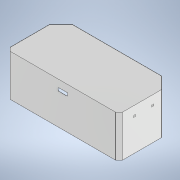
# Autodesk Inventor part: Carcasa
Saved by Autodesk Inventor 2022.1 (Build 261234000, 234)
## iProperties
Created: 2021-10-13
Part Number: Carcasa
Material: PVC, no plastificado
Document SubType Name: Modeling
Designer: seb_0
Density: 1.29 g/cm^3
Appearance: Suave - Blanco
Author: seb_0
Autodesk Inventor part; units mm, degrees
ref_plane "YZ Plane" through (0, 0, 0) normal (1, 0, 0) x (0, 1, 0)
ref_plane "XZ Plane" through (0, 0, 0) normal (0, 1, 0) x (-1, 0, 0)
ref_plane "Plano de trabajo1" through (0, 15.93, 0) normal (0, 0, 1) x (1, 0, 0)
sketch "Boceto1" plane through (0, 15.93, 0) normal (0, 0, 1) x (1, 0, 0)
  line L0 (225, 372.2908) -> (225, -4.1508) projected
  line L1 (224.6622, -4.9663) -> (193.0363, -36.5922) projected
  line L2 (113.0363, 484.7322) -> (224.6622, 373.1063) projected
  line L3 (-744.2208, 485.07) -> (112.2208, 485.07) projected
  line L4 (-857, -4.1508) -> (-857, 372.2908) projected
  line L5 (-825.0363, -36.5922) -> (-856.6622, -4.9663) projected
  line L6 (-856.6622, 373.1063) -> (-745.0363, 484.7322) projected
  line L7 (224.6622, 373.1063) -> (225, 372.2908)
  line L8 (112.2208, 485.07) -> (113.0363, 484.7322)
  line L9 (225, -4.1508) -> (224.6622, -4.9663)
  line L10 (192.2208, -36.93) -> (-824.2208, -36.93) projected
  line L11 (192.2208, -36.93) -> (193.0363, -36.5922)
  line L12 (-825.0363, -36.5922) -> (-824.2208, -36.93)
  line L13 (-857, -4.1508) -> (-856.6622, -4.9663)
  line L14 (-857, 372.2908) -> (-856.6622, 373.1063)
  line L15 (-745.0363, 484.7322) -> (-744.2208, 485.07)
  line L16 (-858.5, -4.4491) -> (-860.9339, 1.4267)
  line L17 (-824.5191, -38.43) -> (192.5191, -38.43)
  line L18 (192.5191, -38.43) -> (193.886, -37.8639)
  line L19 (193.886, -37.8639) -> (225.9339, -5.816)
  line L20 (225.9339, -5.816) -> (226.5, -4.4491)
  line L21 (226.5, -4.4491) -> (226.5, 372.5891)
  line L22 (226.5, 372.5891) -> (225.9339, 373.956)
  line L23 (225.9339, 373.956) -> (113.886, 486.0039)
  line L24 (113.886, 486.0039) -> (112.5191, 486.57)
  line L25 (112.5191, 486.57) -> (-744.5191, 486.57)
  line L26 (-744.5191, 486.57) -> (-745.886, 486.0039)
  line L27 (-745.886, 486.0039) -> (-857.9339, 373.956)
  line L28 (-857.9339, 373.956) -> (-858.5, 372.5891)
  line L29 (-858.5, 372.5891) -> (-858.5, -4.4491)
  line L30 (-858.5, -4.4491) -> (-857.9339, -5.816)
  line L31 (-857.9339, -5.816) -> (-825.886, -37.8639)
  line L32 (-825.886, -37.8639) -> (-824.5191, -38.43)
  point P0 (0, -15.93)
  dimension "d63" = 1.5
  constraints: 50 end point, 8 perpendicular, 15 other
  measures "d63" distance between parallel lines of L10 L17
extrude "Extrusión1" add sketch "Boceto1" against normal blind 400
sketch "Boceto2" plane through (0, 15.93, 0) normal (0, 0, 1) x (1, 0, 0)
  line L0 (-857, -4.1508) -> (-857, 372.2908)
  line L1 (-857, 372.2908) -> (-856.6622, 373.1063)
  line L2 (-856.6622, 373.1063) -> (-745.0363, 484.7322)
  line L3 (-745.0363, 484.7322) -> (-744.2208, 485.07)
  line L4 (-744.2208, 485.07) -> (112.2208, 485.07)
  line L5 (112.2208, 485.07) -> (113.0363, 484.7322)
  line L6 (113.0363, 484.7322) -> (224.6622, 373.1063)
  line L7 (224.6622, 373.1063) -> (225, 372.2908)
  line L8 (225, 372.2908) -> (225, -4.1508)
  line L9 (225, -4.1508) -> (224.6622, -4.9663)
  line L10 (224.6622, -4.9663) -> (193.0363, -36.5922)
  line L11 (-825.0363, -36.5922) -> (-856.6622, -4.9663)
  line L12 (-825.0363, -36.5922) -> (-856.6622, -4.9663)
  line L13 (224.6622, -4.9663) -> (193.0363, -36.5922)
  line L14 (192.2208, -36.93) -> (-824.2208, -36.93)
  line L15 (-857, -4.1508) -> (-857, 372.2908)
  line L16 (193.0363, -36.5922) -> (192.2208, -36.93)
  line L17 (192.2208, -36.93) -> (-824.2208, -36.93)
  line L18 (-824.2208, -36.93) -> (-825.0363, -36.5922)
  line L19 (-825.0363, -36.5922) -> (-856.6622, -4.9663)
  line L20 (-856.6622, -4.9663) -> (-857, -4.1508)
  line L21 (112.5191, 486.57) -> (-744.5191, 486.57)
  line L22 (-825.886, -37.8639) -> (-824.5191, -38.43)
  line L23 (-824.5191, -38.43) -> (192.5191, -38.43)
  line L24 (192.5191, -38.43) -> (193.886, -37.8639)
  line L25 (193.886, -37.8639) -> (225.9339, -5.816)
  line L26 (225.9339, -5.816) -> (226.5, -4.4491)
  line L27 (226.5, -4.4491) -> (226.5, 372.5891)
  line L28 (226.5, 372.5891) -> (225.9339, 373.956)
  line L29 (225.9339, 373.956) -> (113.886, 486.0039)
  line L30 (113.886, 486.0039) -> (112.5191, 486.57)
  line L31 (112.5191, 486.57) -> (-744.5191, 486.57)
  line L32 (-744.5191, 486.57) -> (-745.886, 486.0039)
  line L33 (-745.886, 486.0039) -> (-857.9339, 373.956)
  line L34 (-857.9339, 373.956) -> (-858.5, 372.5891)
  line L35 (-858.5, 372.5891) -> (-858.5, -4.4491)
  line L36 (-858.5, -4.4491) -> (-857.9339, -5.816)
  line L37 (-857.9339, -5.816) -> (-825.886, -37.8639)
  line L38 (-857, -4.1508) -> (-857, 372.2908)
  line L39 (-857, 372.2908) -> (-856.6622, 373.1063)
  line L40 (-856.6622, 373.1063) -> (-745.0363, 484.7322)
  line L41 (-745.0363, 484.7322) -> (-744.2208, 485.07)
  line L42 (-744.2208, 485.07) -> (112.2208, 485.07)
  line L43 (112.2208, 485.07) -> (113.0363, 484.7322)
  line L44 (113.0363, 484.7322) -> (224.6622, 373.1063)
  line L45 (224.6622, 373.1063) -> (225, 372.2908)
  line L46 (225, 372.2908) -> (225, -4.1508)
  line L47 (225, -4.1508) -> (224.6622, -4.9663)
  line L48 (224.6622, -4.9663) -> (193.0363, -36.5922)
  line L49 (193.0363, -36.5922) -> (192.2208, -36.93)
  line L50 (192.2208, -36.93) -> (-824.2208, -36.93)
  line L51 (-824.2208, -36.93) -> (-825.0363, -36.5922)
  line L52 (-825.0363, -36.5922) -> (-856.6622, -4.9663)
  line L53 (-856.6622, -4.9663) -> (-857, -4.1508)
  point P0 (-824.2208, -36.93)
extrude "Extrusión2" add sketch "Boceto2" along normal blind 1.5 contours L0 L1 L2 L3 L4 L5 L6 L7 L8 L9 L10 L16 L14 L18 L11 L20 | L30 L29 L28 L27 L26 L25 L24 L23 L22 L37 L36 L35 L34 L33 L32 L21
sketch "Boceto4" plane through (-744.5191, 502.5, -400) normal (0, 1, 0) x (1, 0, 0)
  line L0 (855.1466, -300) -> (1.8917, -300) projected
  circle A0 centre (655.1466, -310) radius 2.5
  circle A1 centre (201.8917, -310) radius 2.5
  point P0 (744.5191, -400)
  dimension "d5" = 10
  dimension "d6" = 10
  dimension "d7" = 5
  dimension "d8" = 200
  dimension "d9" = 200
  constraints: 2 centre point, 1 equal radius
  measures "d5" distance from line of L0 A0.centre
  measures "d6" distance from line of L0 A1.centre
  measures "d7" diameter of A0
  measures "d8" horizontal distance of L0.start A0.centre
  measures "d9" horizontal distance of A1.centre L0.end
hole "Agujero1" at (-89.3726, 502.5, -90) at (-542.6274, 502.5, -90) direction (0, -1, 0) diameter 3.4 depth 6 tip angle 118 clearance for "Tornillo para maquinaria de cabeza plana" size "M3" standard "Perfil M métrico ANSI"
sketch "Boceto6" plane through (-744.2208, 501, -400) normal (0, -1, 0) x (1, 0, 0)
  circle A0 centre (654.8482, 310) radius 1.7 projected
  circle A1 centre (201.5934, 310) radius 1.7 projected
  circle A2 centre (654.8482, 310) radius 9.2
  circle A3 centre (201.5934, 310) radius 9.2
  line L0 (664.0482, 300.8) -> (645.6482, 300.8)
  line L1 (645.6482, 300.8) -> (645.6482, 319.2)
  line L2 (645.6482, 319.2) -> (664.0482, 319.2)
  line L3 (664.0482, 319.2) -> (664.0482, 300.8)
  line L4 (210.7934, 300.8) -> (192.3934, 300.8)
  line L5 (192.3934, 300.8) -> (192.3934, 319.2)
  line L6 (192.3934, 319.2) -> (210.7934, 319.2)
  line L7 (210.7934, 319.2) -> (210.7934, 300.8)
  point P0 (744.2208, 400)
  dimension "d17" = 7.5
  constraints: 16 end point, 8 tangent, 4 parallel, 2 centre point, 2 horizontal, 2 perpendicular, 1 equal radius
  measures "d17" radial gap between concentric circles of A0 A2
extrude "Extrusión3" add sketch "Boceto6" along normal blind 15
sketch "Boceto7" plane through (-858.5, 27.4109, -400) normal (-1, 0, 0) x (0, 0, 1)
  line L0 (264, 376.8034) -> (264, 0.2349) projected
  circle A0 centre (310, 276.8034) radius 2.5
  circle A1 centre (310, 100.2349) radius 2.5
  line L1 (300, 359.2166) -> (300, -14.0383) projected
  point P0 (400, -27.4109)
  dimension "d21" = 5
  dimension "d23" = 100
  dimension "d24" = 100
  dimension "d60" = 10
  dimension "d62" = 10
  constraints: 2 centre point, 1 equal radius
  measures "d21" diameter of A0
  measures "d23" vertical distance of L0.start A0.centre
  measures "d24" vertical distance of L0.end A1.centre
  measures "d60" distance from line of L1 A0.centre
  measures "d62" distance from line of L1 A1.centre
hole "Agujero2" at (-858.5, 304.2143, -90) at (-858.5, 127.6457, -90) direction (1, 0, 0) diameter 3.4 end through all clearance for "Tornillo para maquinaria de cabeza plana" size "M3" standard "Perfil M métrico ANSI"
sketch "Boceto11" plane through (-744.2208, 486, -400) normal (0, -1, 0) x (1, 0, 0)
  circle A0 centre (201.5934, 310) radius 1.7 projected
  line L0 (204.3434, 308.4123) -> (201.5934, 306.8246)
  line L1 (201.5934, 306.8246) -> (198.8434, 308.4123)
  line L2 (198.8434, 308.4123) -> (198.8434, 311.5877)
  line L3 (198.8434, 311.5877) -> (201.5934, 313.1754)
  line L4 (201.5934, 313.1754) -> (204.3434, 311.5877)
  line L5 (204.3434, 311.5877) -> (204.3434, 308.4123)
  circle A1 centre (654.8482, 310) radius 1.7 projected
  line L6 (657.5982, 308.4123) -> (654.8482, 306.8246)
  line L7 (654.8482, 306.8246) -> (652.0982, 308.4123)
  line L8 (652.0982, 308.4123) -> (652.0982, 311.5877)
  line L9 (652.0982, 311.5877) -> (654.8482, 313.1754)
  line L10 (654.8482, 313.1754) -> (657.5982, 311.5877)
  line L11 (657.5982, 311.5877) -> (657.5982, 308.4123)
  point P0 (744.2208, 400)
  point P1 (201.5934, 310)
  point P2 (654.8482, 310)
  dimension "d39" = 5.5
  dimension "d40" = 5.5
  constraints: 24 end point, 2 coincident, 2 vertical, 26 other
  measures "d39" distance between parallel lines of L2 L5
  measures "d40" distance between parallel lines of L11 L8
extrude "Extrusión6" cut sketch "Boceto11" against normal blind 10
sketch "Boceto12" plane through (-857, 11.7792, -400) normal (1, 0, 0) x (0, 0, -1)
  circle A0 centre (-310, 115.8665) radius 1.7 projected
  circle A1 centre (-310, 292.4351) radius 1.7 projected
  circle A2 centre (-310, 115.8665) radius 9.2
  circle A3 centre (-310, 292.4351) radius 9.2
  line L0 (-319.2, 106.6665) -> (-300.8, 106.6665)
  line L1 (-300.8, 106.6665) -> (-300.8, 125.0665)
  line L2 (-300.8, 125.0665) -> (-319.2, 125.0665)
  line L3 (-319.2, 125.0665) -> (-319.2, 106.6665)
  line L4 (-319.2, 283.2351) -> (-300.8, 283.2351)
  line L5 (-300.8, 283.2351) -> (-300.8, 301.6351)
  line L6 (-300.8, 301.6351) -> (-319.2, 301.6351)
  line L7 (-319.2, 301.6351) -> (-319.2, 283.2351)
  point P0 (-400, -11.7792)
  dimension "d43" = 7.5
  dimension "d44" = 7.5
  constraints: 16 end point, 7 tangent, 4 parallel, 2 centre point, 2 horizontal, 2 perpendicular, 1 point on line
  measures "d43" radial gap between concentric circles of A0 A2
  measures "d44" radial gap between concentric circles of A1 A3
extrude "Extrusión7" add sketch "Boceto12" along normal blind 15
sketch "Boceto13" plane through (-842, 11.7792, -400) normal (1, 0, 0) x (0, 0, -1)
  circle A0 centre (-310, 292.4351) radius 1.7 projected
  circle A1 centre (-310, 115.8665) radius 1.7 projected
  line L0 (-308.4123, 118.6165) -> (-306.8246, 115.8665)
  line L1 (-306.8246, 115.8665) -> (-308.4123, 113.1165)
  line L2 (-308.4123, 113.1165) -> (-311.5877, 113.1165)
  line L3 (-311.5877, 113.1165) -> (-313.1754, 115.8665)
  line L4 (-313.1754, 115.8665) -> (-311.5877, 118.6165)
  line L5 (-311.5877, 118.6165) -> (-308.4123, 118.6165)
  line L6 (-308.4123, 295.1851) -> (-306.8246, 292.4351)
  line L7 (-306.8246, 292.4351) -> (-308.4123, 289.6851)
  line L8 (-308.4123, 289.6851) -> (-311.5877, 289.6851)
  line L9 (-311.5877, 289.6851) -> (-313.1754, 292.4351)
  line L10 (-313.1754, 292.4351) -> (-311.5877, 295.1851)
  line L11 (-311.5877, 295.1851) -> (-308.4123, 295.1851)
  point P0 (-400, -11.7792)
  dimension "d47" = 5.5
  dimension "d48" = 5.5
  constraints: 24 end point, 3 coincident, 2 horizontal, 26 other
  measures "d47" distance between parallel lines of L11 L8
  measures "d48" distance between parallel lines of L2 L5
extrude "Extrusión8" cut sketch "Boceto13" against normal blind 10 contours A0 | L0 L1 L2 L3 L4 L5 | L6 L7 L8 L9 L10 L11
sketch "Boceto14" plane through (225, 11.7792, -400) normal (-1, 0, 0) x (0, 0, 1)
  circle A0 centre (310, 292.4351) radius 1.7 projected
  circle A1 centre (310, 115.8665) radius 1.7 projected
  circle A2 centre (310, 292.4351) radius 9.2
  circle A3 centre (310, 115.8665) radius 9.2
  line L0 (319.2, 301.6351) -> (300.8, 301.6351)
  line L1 (300.8, 301.6351) -> (300.8, 283.2351)
  line L2 (300.8, 283.2351) -> (319.2, 283.2351)
  line L3 (319.2, 283.2351) -> (319.2, 301.6351)
  line L4 (319.2, 125.0665) -> (300.8, 125.0665)
  line L5 (300.8, 125.0665) -> (300.8, 106.6665)
  line L6 (300.8, 106.6665) -> (319.2, 106.6665)
  line L7 (319.2, 106.6665) -> (319.2, 125.0665)
  point P0 (400, -11.7792)
  dimension "d51" = 7.5
  dimension "d52" = 7.5
  constraints: 16 end point, 8 tangent, 4 parallel, 2 centre point, 2 horizontal, 2 perpendicular
  measures "d51" radial gap between concentric circles of A0 A2
  measures "d52" radial gap between concentric circles of A1 A3
extrude "Extrusión9" add sketch "Boceto14" along normal blind 15
sketch "Boceto15" plane through (210, 11.7792, -400) normal (-1, 0, 0) x (0, 0, 1)
  circle A0 centre (310, 292.4351) radius 1.7 projected
  circle A1 centre (310, 115.8665) radius 1.7 projected
  line L0 (308.4123, 289.6851) -> (306.8246, 292.4351)
  line L1 (306.8246, 292.4351) -> (308.4123, 295.1851)
  line L2 (308.4123, 295.1851) -> (311.5877, 295.1851)
  line L3 (311.5877, 295.1851) -> (313.1754, 292.4351)
  line L4 (313.1754, 292.4351) -> (311.5877, 289.6851)
  line L5 (311.5877, 289.6851) -> (308.4123, 289.6851)
  line L6 (308.4123, 113.1165) -> (306.8246, 115.8665)
  line L7 (306.8246, 115.8665) -> (308.4123, 118.6165)
  line L8 (308.4123, 118.6165) -> (311.5877, 118.6165)
  line L9 (311.5877, 118.6165) -> (313.1754, 115.8665)
  line L10 (313.1754, 115.8665) -> (311.5877, 113.1165)
  line L11 (311.5877, 113.1165) -> (308.4123, 113.1165)
  point P0 (400, -11.7792)
  point P1 (310, 292.4351)
  dimension "d55" = 5.5
  dimension "d56" = 5.5
  constraints: 24 end point, 2 coincident, 2 horizontal, 26 other
  measures "d55" distance between parallel lines of L11 L8
  measures "d56" distance between parallel lines of L2 L5
extrude "Extrusión10" cut sketch "Boceto15" against normal blind 10
sketch "Boceto16" plane through (-744.5191, 502.5, -400) normal (0, 1, 0) x (1, 0, 0)
  line L0 (855.8034, -296) -> (-0.7651, -296)
  line L1 (854.1466, -300) -> (0.8917, -300)
  line L2 (468.5191, -300) -> (468.5191, -380)
  line L3 (468.5191, -380) -> (388.5191, -380)
  line L4 (388.5191, -380) -> (388.5191, -300)
  line L5 (80, -300) -> (80, -380)
  line L6 (80, -380) -> (0, -380)
  line L7 (777.0383, -300) -> (777.0383, -380)
  line L8 (857.0383, 0) -> (857.0383, -401.5) projected
  line L9 (0, 0) -> (0, -401.5) projected
  line L10 (777.0383, -380) -> (857.0383, -380)
  line L11 (857.0383, -380) -> (857.0383, -300)
  line L12 (854.1466, -300) -> (857.0383, -300)
  line L13 (0.8917, -300) -> (0, -300)
  line L14 (0, -380) -> (0, -300)
  line L15 (-1.3668, 0) -> (-1.3668, -401.5) projected
  line L16 (777.0383, -380) -> (468.5191, -380)
  line L17 (388.5191, -380) -> (80, -380)
  point P0 (744.5191, -400)
  dimension "d65" = 80
  dimension "d69" = 80
  dimension "d70" = 80
  constraints: 30 end point, 9 point on line, 5 horizontal, 4 perpendicular, 3 equal length, 2 parallel, 2 vertical, 1 collinear, 4 other
  measures "d65" distance of L5.start L5.end
  measures "d69" distance of L2.end L3.end
  measures "d70" distance of L5.end L6.end
extrude "Extrusión11" cut sketch "Boceto16" against normal blind 1.5 contours L12 L8 L10 L7 L1 | L2 L3 L4 L1 | L5 L6 L9 L13 L1
sketch "Boceto17" plane through (-824.5191, -22.5, -400) normal (0, -1, 0) x (1, 0, 0)
  line L0 (468.5191, 331.5) -> (548.5191, 331.5)
  line L1 (553.5191, 326.5) -> (553.5191, 306.5)
  line L2 (548.5191, 301.5) -> (468.5191, 301.5)
  line L3 (463.5191, 306.5) -> (463.5191, 326.5)
  line L4 (0, 401.5) -> (1017.0383, 401.5) projected
  line L5 (463.5191, 316.5) -> (0.2984, 316.5)
  line L6 (0.2984, 400) -> (0.2984, 0) projected
  line L7 (553.5191, 316.5) -> (1016.7399, 316.5)
  line L8 (1016.7399, 400) -> (1016.7399, 0) projected
  arc A0 (468.5191, 331.5) -> (463.5191, 326.5) centre (468.5191, 326.5) ccw
  arc A1 (463.5191, 306.5) -> (468.5191, 301.5) centre (468.5191, 306.5) ccw
  arc A2 (548.5191, 301.5) -> (553.5191, 306.5) centre (548.5191, 306.5) ccw
  arc A3 (553.5191, 326.5) -> (548.5191, 331.5) centre (548.5191, 326.5) ccw
  point P0 (824.5191, 400)
  point P1 (463.5191, 331.5)
  point P2 (553.5191, 301.5)
  point P3 (553.5191, 331.5)
  point P4 (463.5191, 301.5)
  dimension "d71" = 70
  dimension "d72" = 30
  dimension "d73" = 90
  dimension "d76" = 5
  dimension "d77" = 5
  dimension "d78" = 5
  dimension "d79" = 5
  constraints: 12 end point, 10 point on line, 8 point on circle, 8 tangent, 4 centre point, 3 horizontal, 2 midpoint, 2 parallel, 1 collinear, 1 perpendicular
  measures "d71" distance between parallel lines of L4 L0
  measures "d72" distance of point (553.519, 331.5) point (553.519, 301.5)
  measures "d73" distance of point (463.519, 331.5) point (553.519, 331.5)
  measures "d76" radius of A0
  measures "d77" radius of A1
  measures "d78" radius of A2
  measures "d79" radius of A3
extrude "Extrusión12" cut sketch "Boceto17" against normal blind 1.5
